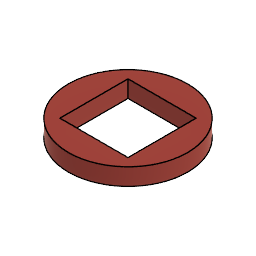
sparation_ring (Autodesk Fusion 360 design; units mm, degrees)
part number: 2026-05-05-03-19-49-403
Autodesk Fusion 360 part; units mm, degrees
sketch "Sketch1" plane through (0, 0, 0) normal (0, 0, 1) x (1, 0, 0)
  circle A0 centre (0, 0) radius 3.5
  line L0 (0, 0) -> (2, 0)
  line L1 (2, 0) -> (2, 2)
  line L2 (2, 2) -> (-2, 2)
  line L3 (-2, 2) -> (-2, -2)
  line L4 (-2, -2) -> (2, -2)
  line L5 (2, -2) -> (2, 0)
  dimension "d1" = 7
  dimension "d2" = 2
  dimension "d3" = 2
  dimension "d4" = 4
  dimension "d5" = 4
  dimension "d6" = 4
  dimension "d7" = 2
  constraint coincident A0.centre L0.start
  constraint horizontal L0
  constraint perpendicular L0 L1
  constraint perpendicular L1 L2
  constraint perpendicular L2 L3
  constraint perpendicular L3 L4
  constraint perpendicular L2 L5
  measures "d1" diameter of A0
  measures "d2" distance of A0.centre L0.end
  measures "d3" distance of L0.end L1.end
  measures "d4" distance of L1.end L2.end
  measures "d5" distance of L2.end L3.end
  measures "d6" distance of L3.end L4.end
  measures "d7" distance of L4.end L0.end
extrude "Extrude1" add sketch "Sketch1" along normal blind 1
equation "d3 = d2"
equation "d4 = d2 * 2"
equation "d5 = d2 * 2"
equation "d6 = d2 * 2"
equation "d7 = d2"
